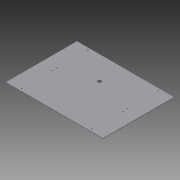
# Autodesk Inventor part: lift plate
Saved by Autodesk Inventor 2015 SP1 (Build 190203100, 203)
## iProperties
Created: 2015-01-13
Part Number: lift plate
Material: Generic
Document SubType Name: Modeling
Designer: Jarod
Density: 1 g/cm^3
Appearance: Default
Author: Jarod
Autodesk Inventor part; units mm, degrees
ref_plane "YZ Plane" through (0, 0, 0) normal (1, 0, 0) x (0, 1, 0)
ref_plane "XZ Plane" through (0, 0, 0) normal (0, 1, 0) x (-1, 0, 0)
ref_plane "XY Plane" through (0, 0, 0) normal (0, 0, 1) x (1, 0, 0)
sketch "Sketch1" plane through (0, 0, 0) normal (0, 1, 0) x (-1, 0, 0)
  line L0 (0, 0) -> (520.7, 0)
  line L1 (520.7, 0) -> (520.7, 381)
  line L2 (520.7, 381) -> (0, 381)
  line L3 (0, 381) -> (0, 0)
  dimension "d0" = 520.7
  dimension "d1" = 381
  constraints: 8 end point, 2 parallel, 1 horizontal, 1 perpendicular
  measures "d0" distance of L2.end L1.end
  measures "d1" distance of L1.end L0.end
extrude "Extrusion1" add sketch "Sketch1" along normal blind 3.175
sketch "Sketch2" plane through (0, 3.175, 0) normal (0, 1, 0) x (1, 0, 0)
  line L0 (0, 0) -> (-520.7, 0) projected
  line L1 (-520.7, 0) -> (-520.7, -381) projected
  line L2 (-520.7, -381) -> (0, -381) projected
  line L3 (0, -381) -> (0, 0) projected
  point P0 (-58.7375, -368.3)
  point P1 (-461.9625, -368.3)
  point P2 (-461.9625, -12.7)
  point P3 (-58.7375, -12.7)
  dimension "d4" = 58.7375
  dimension "d5" = 58.7375
  dimension "d6" = 58.7375
  dimension "d7" = 58.7375
  dimension "d8" = 12.7
  dimension "d9" = 12.7
  dimension "d10" = 12.7
  dimension "d11" = 12.7
  measures "d4" distance from line of L3 point (-58.738, -368.3)
  measures "d5" distance from line of point (-58.738, -12.7) L3
  measures "d6" distance from line of L1 point (-461.962, -368.3)
  measures "d7" distance from line of L1 point (-461.962, -12.7)
  measures "d8" distance from line of L0 point (-461.962, -12.7)
  measures "d9" distance from line of L2 point (-461.962, -368.3)
  measures "d10" distance from line of L2 point (-58.738, -368.3)
  measures "d11" distance from line of L0 point (-58.738, -12.7)
hole "Hole1" at (-58.7375, 3.175, 368.3) at (-461.9625, 3.175, 368.3) at (-461.9625, 3.175, 12.7) at (-58.7375, 3.175, 12.7) direction (0, -1, 0) diameter 6.35 end through all
sketch "Sketch3" plane through (0, 3.175, 0) normal (0, 1, 0) x (1, 0, 0)
  circle A0 centre (-461.9625, -12.7) radius 3.175 projected
  circle A1 centre (-58.7375, -368.3) radius 3.175 projected
  circle A2 centre (-461.9625, -368.3) radius 3.175 projected
  circle A3 centre (-58.7375, -12.7) radius 3.175 projected
  line L0 (0, 0) -> (-520.7, 0) projected
  line L1 (-520.7, 0) -> (-520.7, -381) projected
  line L2 (-520.7, -381) -> (0, -381) projected
  line L3 (0, -381) -> (0, 0) projected
  point P0 (-58.7375, -203.2)
  point P1 (-58.7375, -177.8)
  point P2 (-461.9625, -177.8)
  point P3 (-461.9625, -203.2)
  dimension "d19" = 177.8
  dimension "d20" = 177.8
  dimension "d21" = 177.8
  dimension "d22" = 177.8
  dimension "d23" = 58.7375
  dimension "d24" = 58.7375
  dimension "d25" = 58.7375
  dimension "d26" = 58.7375
  measures "d19" distance from line of L2 point (-58.738, -203.2)
  measures "d20" distance from line of L0 point (-58.738, -177.8)
  measures "d21" distance from line of L2 point (-461.962, -203.2)
  measures "d22" distance from line of L0 point (-461.962, -177.8)
  measures "d23" distance from line of L1 point (-461.962, -203.2)
  measures "d24" distance from line of L1 point (-461.962, -177.8)
  measures "d25" distance from line of point (-58.738, -177.8) L3
  measures "d26" distance from line of L3 point (-58.738, -203.2)
hole "Hole2" at (-58.7375, 3.175, 203.2) at (-58.7375, 3.175, 177.8) at (-461.9625, 3.175, 177.8) at (-461.9625, 3.175, 203.2) direction (0, -1, 0) diameter 6.35 end through all
sketch "Sketch4" plane through (0, 3.175, 0) normal (0, 1, 0) x (1, 0, 0)
  circle A0 centre (-461.9625, -177.8) radius 3.175 projected
  circle A1 centre (-58.7375, -203.2) radius 3.175 projected
  circle A2 centre (-58.7375, -177.8) radius 3.175 projected
  circle A3 centre (-461.9625, -203.2) radius 3.175 projected
  circle A4 centre (-461.9625, -12.7) radius 3.175 projected
  circle A5 centre (-58.7375, -368.3) radius 3.175 projected
  circle A6 centre (-461.9625, -368.3) radius 3.175 projected
  circle A7 centre (-58.7375, -12.7) radius 3.175 projected
  line L0 (0, 0) -> (-520.7, 0) projected
  line L1 (-520.7, 0) -> (-520.7, -381) projected
  line L2 (-520.7, -381) -> (0, -381) projected
  line L3 (0, -381) -> (0, 0) projected
  circle A8 centre (-260.35, -127) radius 9.525
  line L4 (-260.35, -127) -> (-278.3105, -144.9605) construction
  line L5 (-260.35, -127) -> (-234.95, -127) construction
  line L6 (-260.35, -127) -> (-242.3895, -109.0395) construction
  line L7 (-260.35, -127) -> (-234.95, -127) construction
  circle A9 centre (-278.3105, -144.9605) radius 1.9844
  circle A10 centre (-242.3895, -109.0395) radius 1.9844
  dimension "d34" = 19.05
  dimension "d35" = 127
  dimension "d36" = 260.35
  dimension "d37" = 25.4
  dimension "d38" = 135
  dimension "d39" = 25.4
  dimension "d40" = 45
  dimension "d41" = 3.9688
  dimension "d42" = 3.9688
  constraints: 8 end point, 3 centre point, 2 coincident, 2 equal length, 2 horizontal
  measures "d34" diameter of A8
  measures "d35" distance from line of L0 L4.start
  measures "d36" distance from line of L4.start L3
  measures "d37" distance of L4.start L4.end
  measures "d38" angle of L4 L5
  measures "d39" distance of L4.start L6.end
  measures "d40" angle of L7 L6
  measures "d41" diameter of A9
  measures "d42" diameter of A10
extrude "Extrusion2" cut sketch "Sketch4" against normal blind 3.175 contours A8 | A9 | A10
body "Solid1"
